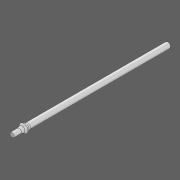
# Autodesk Inventor part: SealantApplicator
Saved by Autodesk Inventor 2020 (Build 240168000, 168)
## iProperties
Created: 2020-01-15
Part Number: SealantApplicator
Material: Generic
Document SubType Name: Modeling
Designer: Isaac Newcomb
Density: 1 g/cm^3
Appearance: Default
Author: Isaac Newcomb
Autodesk Inventor part; units mm, degrees
ref_plane "YZ Plane" through (0, 0, 0) normal (1, 0, 0) x (0, 1, 0)
ref_plane "XZ Plane" through (0, 0, 0) normal (0, 1, 0) x (-1, 0, 0)
ref_plane "XY Plane" through (0, 0, 0) normal (0, 0, 1) x (1, 0, 0)
sketch "Sketch1" plane through (0, 0, 0) normal (0, 1, 0) x (-1, 0, 0)
  line L0 (-3, -16.9821) -> (-3, -180)
  line L1 (-3, -180) -> (0, -180)
  line L2 (0, -180) -> (0, 0)
  line L3 (-5, -13.3299) -> (0, -13.3299) construction
  line L4 (-5, -13.3299) -> (-5, -15.3949) construction
  line L5 (-3, -16.9821) -> (-5, -13.3299)
  line L6 (-5, -13.3299) -> (-2.5, -10)
  line L7 (-2.5, -10) -> (-2.5, 0)
  line L8 (-2.5, 0) -> (0, 0)
  dimension "d5" = 180
  dimension "d8" = 5
  dimension "d12" = 6
  dimension "d14" = 10
  dimension "d15" = 7
  dimension "d16" = 5
  constraints: 19 end point, 3 perpendicular, 3 vertical, 1 equal length, 1 horizontal, 1 point on line
  measures "d5" distance of L1.end L2.end
  measures "d8" distance of L3.start L3.end
  measures "d12" diameter of L0 L2
  measures "d14" distance of L6.end L7.end
  measures "d15" distance of L0.start L6.end
  measures "d16" diameter of L7 L2
revolve "Revolution1" add sketch "Sketch1" angle 360 about axis through (0, 0, -180) along (0, 0, 1)
fillet "Fillet2" radius 5 2 edges at (-3, 0, -16.9821) (-2.5, 0, -10)
body "Solid1"
